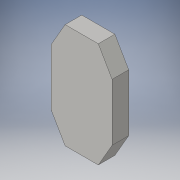
# Autodesk Inventor part: 4901BaseSolidGeometry
Saved by Autodesk Inventor 2016 (Build 200138000, 138)
## iProperties
Created: 2016-01-14
Part Number: 4901BaseSolidGeometry
Material: Generic
Document SubType Name: Modeling
Designer: ryann
Density: 1 g/cm^3
Appearance: Default
Author: ryann
Autodesk Inventor part; units mm, degrees
ref_plane "YZ Plane" through (0, 0, 0) normal (1, 0, 0) x (0, 1, 0)
ref_plane "XZ Plane" through (0, 0, 0) normal (0, 1, 0) x (-1, 0, 0)
ref_plane "XY Plane" through (0, 0, 0) normal (0, 0, 1) x (1, 0, 0)
sketch "Sketch1" plane through (0, 0, 0) normal (0, 0, 1) x (1, 0, 0)
  point P0 (0, 0)
sketch "Sketch2" plane through (0, 0, 0) normal (0, 0, 1) x (1, 0, 0)
  line L0 (127, 965.2) -> (341.7889, 965.2) construction
  line L1 (279.4, 965.2) -> (279.4, 0) construction
  line L2 (279.4, 482.6) -> (-286.2053, 482.6) construction
  line L3 (127, 965.2) -> (0, 745.2295)
  line L4 (431.8, 965.2) -> (558.8, 745.2295)
  line L5 (127, 0) -> (0, 219.9705)
  line L6 (431.8, 0) -> (558.8, 219.9705)
  line L7 (0, 219.9705) -> (0, 745.2295)
  line L8 (558.8, 745.2295) -> (558.8, 219.9705)
  line L9 (0, 745.2295) -> (127, 965.2)
  line L10 (0, 745.2295) -> (0, 219.9705)
  line L11 (0, 219.9705) -> (127, 0)
  line L12 (431.8, 0) -> (558.8, 219.9705)
  line L13 (558.8, 219.9705) -> (558.8, 745.2295)
  line L14 (558.8, 745.2295) -> (431.8, 965.2)
  line L15 (127, 0) -> (431.8, 0)
  line L16 (431.8, 965.2) -> (127, 965.2)
  point P0 (0, 0)
  point P1 (341.7889, 0)
  dimension "d3" = 152.4
  dimension "d4" = 152.4
  dimension "d10" = 525.2591
  dimension "d11" = 525.2591
  dimension "d15" = 304.8
  dimension "d16" = 219.9704
  constraints: 34 end point, 6 symmetric about line, 5 collinear, 3 vertical, 2 horizontal, 1 midpoint, 1 parallel
  measures "d3" distance of L1.start L0.start
  measures "d4" distance of L1.start L4.start
  measures "d10" distance of L4.end L8.end
  measures "d11" distance of L5.end L7.end
  measures "d15" distance of L6.start L5.start
  measures "d16" distance from line of L15 L6.end
extrude "Extrusion1" add sketch "Sketch2" along normal blind 152.4
body "Solid1"
